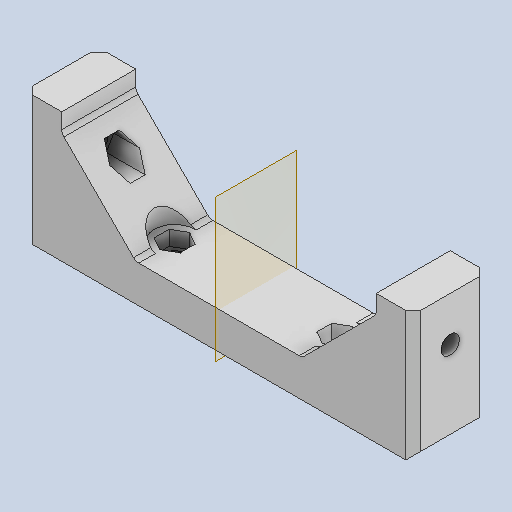
# Autodesk Inventor part: BatteryHolderSide
Saved by Autodesk Inventor 2022 (Build 260153000, 153)
## iProperties
Created: 2021-02-16
Part Number: BatteryHolderSide
Material: Generic
Document SubType Name: Modeling
Designer: Viktor
Density: 1 g/cm^3
Appearance: Default
Author: Viktor
## iProperties of the stored document _3DPrint.ipt
Created: 2021-02-17
Part Number: _3DPrint
Material: Generic
Document SubType Name: Modeling
Designer: Viktor
Density: 1 g/cm^3
Appearance: Default
Author: Viktor
Autodesk Inventor part; units mm, degrees
ref_plane "XZ Plane" through (0, 0, 0) normal (0, 1, 0) x (-1, 0, 0)
ref_plane "XY Plane" through (0, 0, 0) normal (0, 0, 1) x (1, 0, 0)
sketch "Sketch1" plane through (0, 0, 0) normal (0, 0, 1) x (1, 0, 0)
  line L0 (-52.5, -17.5) -> (52.5, -17.5)
  line L1 (52.5, -17.5) -> (52.5, 17.5)
  line L2 (52.5, 17.5) -> (-52.5, 17.5)
  line L3 (-52.5, 17.5) -> (-52.5, -17.5)
  line L4 (-52.5, -17.5) -> (52.5, 17.5) construction
  line L5 (52.5, -17.5) -> (-52.5, 17.5) construction
  point P0 (0, 0)
  dimension "d0" = 105
  dimension "d1" = 35
  constraints: 12 end point, 2 midpoint, 2 parallel, 1 horizontal, 1 perpendicular
  measures "d0" distance between parallel lines of L1 L3
  measures "d1" distance between parallel lines of L0 L2
extrude "Extrusion1" add sketch "Sketch1" along normal blind 20
sketch "Sketch2" plane through (0, 0, 20) normal (0, 0, 1) x (1, 0, 0)
  line L0 (52.5, 17.5) -> (-52.5, 17.5) projected
  line L1 (-42.5, 17.5) -> (42.5, 17.5)
  line L2 (42.5, 17.5) -> (42.5, -7.5)
  line L3 (42.5, -7.5) -> (-42.5, -7.5)
  line L4 (-42.5, -7.5) -> (-42.5, 17.5)
  line L5 (-52.5, 17.5) -> (-52.5, -17.5) projected
  line L6 (52.5, -17.5) -> (52.5, 17.5) projected
  line L7 (-52.5, -17.5) -> (52.5, -17.5) projected
  point P0 (0, 0)
  point P1 (42.5, 17.5)
  dimension "d4" = 10
  dimension "d5" = 10
  dimension "d6" = 10
  constraints: 8 end point, 2 parallel, 1 horizontal, 1 perpendicular, 1 point on line
  measures "d4" distance between parallel lines of L5 L4
  measures "d5" distance between parallel lines of L6 L2
  measures "d6" distance between parallel lines of L7 L3
extrude "Extrusion2" cut sketch "Sketch2" against normal through all contours L2 L3 L4 L0
chamfer "Chamfer1" distance 20 angle 45 2 edges at (-42.5, -7.5, 10) (42.5, -7.5, 10)
fillet "Fillet1" radius 2 4 edges at (-42.5, 12.5, 10) (-22.5, -7.5, 10) (22.5, -7.5, 10) (42.5, 12.5, 10)
sketch "Sketch3" plane through (-21.6716, -7.5, 20) normal (0, 1, 0) x (1, 0, 0)
  line L0 (-35.2748, 10) -> (83.1656, 10) construction
  circle A0 centre (-0.3284, 10) radius 2.5
  line L1 (21.6716, 24) -> (21.6716, -4) projected
  circle A1 centre (43.6716, 10) radius 2.5
  point P0 (21.6716, 20)
  dimension "d13" = 5
  dimension "d14" = 22
  constraints: 2 centre point, 2 end point, 1 horizontal, 1 point on line, 1 symmetric about line, 1 other
  measures "d13" diameter of A0
  measures "d14" distance from line of L1 A0.centre
extrude "Extrusion3" cut sketch "Sketch3" against normal through all both and the other way through all
sketch "Sketch4" plane through (-21.6716, -7.5, 20) normal (0, 1, 0) x (1, 0, 0)
  arc A0 (-1.4142, 12.2519) -> (-1.4142, 7.7481) centre (-0.3284, 10) ccw projected
  arc A1 (44.7574, 7.7481) -> (44.7574, 12.2519) centre (43.6716, 10) ccw projected
  circle A2 centre (-0.3284, 10) radius 5.5
  circle A3 centre (43.6716, 10) radius 5.5
  point P0 (21.6716, 20)
  dimension "d17" = 11
  dimension "d18" = 11
  constraints: 2 centre point, 2 coincident
  measures "d17" diameter of A2
  measures "d18" diameter of A3
extrude "Extrusion4" cut sketch "Sketch4" along normal blind 20
sketch "Sketch5" plane through (52.5, -17.5, 0) normal (1, 0, 0) x (0, 0, -1)
  circle A0 centre (-10, 23) radius 2.5
  line L0 (-20, 0) -> (-20, 35) projected
  line L1 (0, 35) -> (-20, 35) projected
  point P0 (0, 17.5)
  dimension "d21" = 10
  dimension "d22" = 12
  dimension "d23" = 5
  constraints: 1 centre point
  measures "d21" distance from line of L0 A0.centre
  measures "d22" distance from line of L1 A0.centre
  measures "d23" diameter of A0
extrude "Extrusion5" cut sketch "Sketch5" against normal through all
chamfer "Chamfer2" distance 2 angle 45 6 edges at (-52.5, 0, 20) (-52.5, 0, 0) (52.5, 0, 20) (52.5, 0, 0) (-52.5, -17.5, 10) (52.5, -17.5, 10)
sketch "Sketch6" plane through (-42.5, 17.5, 20) normal (1, 0, 0) x (0, 0, -1)
  circle A0 centre (10, -12) radius 2.5 projected
  circle A1 centre (10, -12) radius 5.5
  point P0 (20, -17.5)
  dimension "d29" = 11
  constraints: 1 centre point
  measures "d29" diameter of A1
extrude "Extrusion6" cut sketch "Sketch6" along normal blind 20
mirror "Mirror1" about plane through (0, 0, 0) normal (1, 0, 0) of "Extrusion6"
sketch "Sketch7" plane through (-42.5, 5.5, 10) normal (1, 0, 0) x (0, 0, -1)
  circle A0 centre (0, 0) radius 5.5 projected
  line L0 (4.0415, 0) -> (2.0207, -3.5)
  line L1 (2.0207, -3.5) -> (-2.0207, -3.5)
  line L2 (-2.0207, -3.5) -> (-4.0415, 0)
  line L3 (-4.0415, 0) -> (-2.0207, 3.5)
  line L4 (-2.0207, 3.5) -> (2.0207, 3.5)
  line L5 (2.0207, 3.5) -> (4.0415, 0)
  point P0 (10, -5.5)
  dimension "d32" = 7
  constraints: 12 end point, 1 coincident, 1 horizontal, 13 other
  measures "d32" distance between parallel lines of L1 L4
extrude "Extrusion7" add sketch "Sketch7" along normal up to surface surface through (-32.5, 2.5, 20) normal (0.7071, 0.7071, 0)
sketch "Sketch8" plane through (-21.6716, -7.5, 20) normal (0, 1, 0) x (1, 0, 0)
  arc A0 (-1.4142, 15.3918) -> (-1.4142, 4.6082) centre (-0.3284, 10) ccw projected
  circle A1 centre (-0.3284, 10) radius 5.5
  line L0 (-0.3284, 14.0415) -> (3.1716, 12.0207)
  line L1 (3.1716, 12.0207) -> (3.1716, 7.9793)
  line L2 (3.1716, 7.9793) -> (-0.3284, 5.9585)
  line L3 (-0.3284, 5.9585) -> (-3.8284, 7.9793)
  line L4 (-3.8284, 7.9793) -> (-3.8284, 12.0207)
  line L5 (-3.8284, 12.0207) -> (-0.3284, 14.0415)
  point P0 (21.6716, 20)
  dimension "d35" = 7
  constraints: 12 end point, 2 coincident, 1 centre point, 1 vertical, 13 other
  measures "d35" distance between parallel lines of L1 L4
extrude "Extrusion8" cut sketch "Sketch8" against normal blind 4 contours L0 L1 L2 L3 L4 L5
mirror "Mirror2" about plane through (0, 0, 0) normal (1, 0, 0) of "Extrusion7", "Extrusion8"
body "Solid1"
